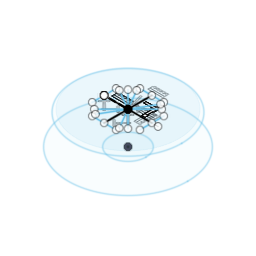
INJECTOR FILE FOR 3D PRINTING(TEST  MODEL 1 ) v1 (Autodesk Fusion 360 design; units mm, degrees)
Autodesk Fusion 360 part; units mm, degrees
sketch "Sketch1" plane through (0, 0, 0) normal (0, 0, 1) x (1, 0, 0)
  circle A0 centre (0, 0) radius 50
  constraint coincident A0.centre origin
extrude "Extrude1" add sketch "Sketch1" along normal blind 30
ref_plane "WorkPlane1" through (0, 0, 25) normal (0, 0, 1) x (1, 0, 0)
sketch "Sketch2" plane through (0, 0, 25) normal (0, 0, 1) x (1, 0, 0)
  circle A0 centre (0, 0) radius 45
extrude "Extrude2" cut sketch "Sketch2" along normal blind 5
sketch "Sketch3" plane through (0, 0, 0) normal (0, 0, 1) x (1, 0, 0)
  circle A0 centre (0, 0) radius 15
  constraint coincident A0.centre origin
sketch "Sketch4" plane through (0, 0, 25) normal (0, 0, 1) x (1, 0, 0)
sketch "Sketch5" plane through (0, 0, 0) normal (1, 0, 0) x (0, 1, 0)
sketch "Sketch6" plane through (0, 0, 0) normal (1, 0, 0) x (0, 1, 0)
sketch "Sketch7" plane through (0, 0, 25) normal (0, 0, 1) x (1, 0, 0)
sketch "Sketch8" plane through (0, 0, 0) normal (1, 0, 0) x (0, 1, 0)
ref_plane "WorkPlane2" through (50, 0, 0) normal (1, 0, 0) x (0, 1, 0)
sketch "Sketch9" plane through (50, 0, 0) normal (1, 0, 0) x (0, 1, 0)
extrude "Extrude3" add sketch "Sketch3" against normal blind 25
sketch "Sketch10" plane through (45, 10, 12.9326) normal (1, 0, 0) x (0, 1, 0)
ref_plane "WorkPlane4" through (51, 0, 0) normal (1, 0, 0) x (0, 1, 0)
sketch "Sketch11" plane through (51, 0, 0) normal (1, 0, 0) x (0, 1, 0)
shell "Shell1" thickness 2.286 outward yes removed faces 1 at (0.9463, -5.6032, -25)
sketch "Sketch12" plane through (0, 0, 0) normal (1, 0, 0) x (0, 1, 0)
ref_plane "WorkPlane5" through (-47, 0, 0) normal (1, 0, 0) x (0, 1, 0)
sketch "Sketch13" plane through (-47, 0, 0) normal (1, 0, 0) x (0, 1, 0)
sketch "Sketch14" plane through (0, 0, 27.286) normal (0, 0, 1) x (-1, 0, 0)
  circle A0 centre (0, 0) radius 42.714
  line L0 (0, 0) -> (-20, 0)
  line L1 (0, 0) -> (0, -20)
  line L2 (0, 0) -> (0, 20)
  line L3 (0, 0) -> (20, 0)
  line L4 (10, -20) -> (-10, -20)
  line L5 (-20, -10) -> (-20, 10)
  line L6 (10, 20) -> (-10, 20)
  line L7 (20, -10) -> (20, 10)
  line L8 (0, 0) -> (-25.164, 0) construction
  line L9 (0, 0) -> (20, 0) construction
  line L10 (0, 0) -> (-14.1421, -14.1421)
  line L11 (0, 0) -> (20, 0) construction
  line L12 (0, 0) -> (14.1421, -14.1421)
  line L13 (0, 0) -> (20, 0) construction
  line L14 (0, 0) -> (-14.1421, 14.1421)
  line L15 (0, 0) -> (20, 0) construction
  line L16 (0, 0) -> (14.1421, 14.1421)
  line L17 (0, 0) -> (20, 0) construction
  line L18 (0, 0) -> (10, -17.3205)
  line L19 (0, 0) -> (20, 0) construction
  line L20 (0, 0) -> (-10, -17.3205)
  line L21 (0, 0) -> (20, 0) construction
  line L22 (0, 0) -> (10, 17.3205)
  line L23 (0, 0) -> (20, 0) construction
  line L24 (0, 0) -> (-10, 17.3205)
  line L25 (0, 0) -> (20, 0) construction
  line L26 (0, 0) -> (17.3205, -10)
  line L27 (0, 0) -> (20, 0) construction
  constraint coincident A0.centre L0.start
  constraint horizontal L0
  constraint perpendicular L0 L1
  constraint perpendicular L0 L2
  constraint perpendicular L2 L3
  constraint horizontal L4
  constraint vertical L5
  constraint perpendicular L2 L6
  constraint perpendicular L3 L7
  constraint horizontal L8
  constraint horizontal L9
  constraint horizontal L11
  constraint perpendicular L10 L12
  constraint horizontal L13
  constraint horizontal L15
  constraint horizontal L17
  constraint perpendicular L14 L16
  constraint horizontal L19
  constraint horizontal L21
  constraint horizontal L23
  constraint horizontal L25
  constraint horizontal L27
  constraint perpendicular L20 L26
hidden bodies 1
